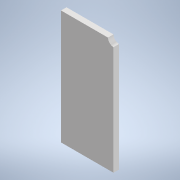
# Autodesk Inventor part: shelf
Saved by Autodesk Inventor 2022 (Build 260153000, 153)
## iProperties
Created: 2022-05-12
Part Number: shelf
Material: Generic
Document SubType Name: Modeling
Designer: Jeanette Guo
Density: 1 g/cm^3
Appearance: Default
Author: Jeanette Guo
Autodesk Inventor part; units mm, degrees
ref_plane "YZ Plane" through (0, 0, 0) normal (1, 0, 0) x (0, 1, 0)
ref_plane "XZ Plane" through (0, 0, 0) normal (0, 1, 0) x (-1, 0, 0)
ref_plane "XY Plane" through (0, 0, 0) normal (0, 0, 1) x (1, 0, 0)
sketch "Sketch1" plane through (0, 0, 0) normal (0, 0, 1) x (1, 0, 0)
  line L0 (60, 32) -> (-60, 32) projected
  line L1 (31.5, 94) -> (31.5, 32) projected
  line L2 (60, -26) -> (60, 94) projected
  line L3 (-63, 94) -> (63, 94) projected
  line L4 (31.5, 94) -> (60, 94)
  line L5 (60, 94) -> (60, 32)
  line L6 (60, 32) -> (31.5, 32)
  line L7 (31.5, 32) -> (31.5, 94)
  line L8 (57, 97) -> (57, 94) projected
  line L9 (57, 97) -> (35, 97)
  line L10 (35, 97) -> (35, 94)
  line L11 (35, 32) -> (35, 29)
  line L12 (35, 29) -> (57, 29)
  line L13 (57, 29) -> (57, 32)
  arc A0 (57, 94) -> (60, 91) centre (60, 94) ccw
  line L14 (57, 94) -> (60, 91) construction
  line L15 (57, 94) -> (61.2426, 94) construction
  point P0 (0, 0)
  point P1 (60, 91)
  point P2 (31.5, 94)
  dimension "d0" = 22
  dimension "d1" = 3
  dimension "d2" = 45
  dimension "d3" = 3
  constraints: 22 end point, 6 point on line, 4 perpendicular, 3 horizontal, 2 parallel, 2 point on circle, 1 centre point, 1 equal length
  measures "d0" distance of L8.start L9.end
  measures "d1" distance of L11.start L11.end
  measures "d2" angle of L14 L15
  measures "d3" radius of A0
extrude "Extrusion1" add sketch "Sketch1" along normal blind 3 contours L0 L1 L3 A0 L2
body "Solid1"
